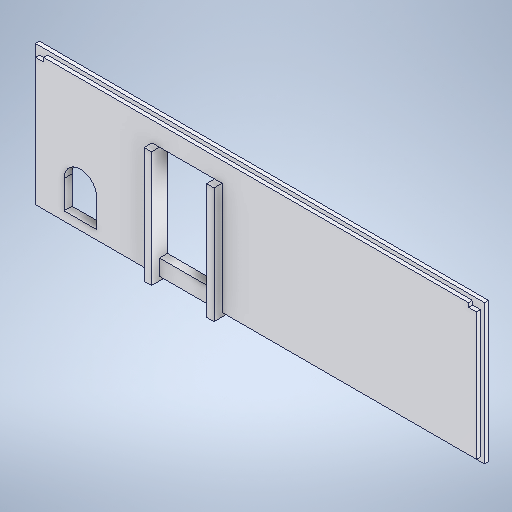
# Autodesk Inventor part: back
Saved by Autodesk Inventor 2025 (Build 290162000, 162)
## iProperties
Created: 2025-05-20
Part Number: back
Material: Generic
Document SubType Name: Modeling
Designer: ethan
Density: 1 g/cm^3
Appearance: PTFE
Author: ethan
Autodesk Inventor part; units mm, degrees
ref_plane "YZ Plane" through (0, 0, 0) normal (1, 0, 0) x (0, 1, 0)
ref_plane "XZ Plane" through (0, 0, 0) normal (0, 1, 0) x (-1, 0, 0)
ref_plane "XY Plane" through (0, 0, 0) normal (0, 0, 1) x (1, 0, 0)
sketch "Sketch1" plane through (0, 0, 0) normal (0, 0, 1) x (1, 0, 0)
  line L0 (0, 0) -> (224.6, 0)
  line L1 (224.6, 0) -> (224.6, 69.85)
  line L2 (224.6, 69.85) -> (0, 69.85)
  line L3 (0, 69.85) -> (0, 0)
  dimension "d0" = 224.6
  dimension "d1" = 69.85
  constraints: 8 end point, 2 parallel, 1 horizontal, 1 perpendicular
  measures "d0" distance of L2.end L1.end
  measures "d1" distance of L1.end L0.end
extrude "Extrusion1" add sketch "Sketch1" along normal blind 2
sketch "Sketch2" plane through (0, 0, 2) normal (0, 0, 1) x (1, 0, 0)
  line L0 (224.6, 0) -> (224.6, 69.85) projected
  line L1 (224.6, 69.85) -> (0, 69.85) projected
  line L2 (0, 69.85) -> (0, 0) projected
  line L3 (0, 0) -> (224.6, 0) projected
  line L4 (2, 67.85) -> (222.6, 67.85)
  line L5 (222.6, 67.85) -> (222.6, 2)
  line L6 (222.6, 2) -> (2, 2)
  line L7 (2, 2) -> (2, 67.85)
  dimension "d4" = 2
  constraints: 8 end point, 3 other
  measures "d4" distance between parallel lines of L1 L4
extrude "Extrusion2" add sketch "Sketch2" along normal blind 2 contours L4 L5 L6 L7
sketch "Sketch3" plane through (0, 0, 4) normal (0, 0, 1) x (1, 0, 0)
  line L0 (2, 2) -> (222.6, 2) construction
  line L1 (222.6, 2) -> (222.6, 67.85) construction
  line L2 (222.6, 67.85) -> (2, 67.85) construction
  line L3 (2, 67.85) -> (2, 2) construction
  line L4 (2, 67.85) -> (6, 67.85)
  line L5 (6, 67.85) -> (6, 65.85)
  line L6 (6, 65.85) -> (2, 65.85)
  line L7 (2, 65.85) -> (2, 67.85)
  line L8 (222.6, 67.85) -> (218.6, 67.85)
  line L9 (218.6, 67.85) -> (218.6, 65.85)
  line L10 (218.6, 65.85) -> (222.6, 65.85)
  line L11 (222.6, 65.85) -> (222.6, 67.85)
  point P0 (0, 0)
  dimension "d7" = 4
  dimension "d8" = 2
  dimension "d9" = 4
  dimension "d10" = 2
  constraints: 16 end point, 4 parallel, 2 horizontal, 2 perpendicular
  measures "d7" distance of L5.end L6.end
  measures "d8" distance of L4.end L5.end
  measures "d9" distance of L10.end L9.end
  measures "d10" distance of L9.end L8.end
extrude "Extrusion3" cut sketch "Sketch3" against normal blind 2
sketch "Sketch4" plane through (0, 0, 4) normal (0, 0, 1) x (1, 0, 0)
  line L0 (6, 67.85) -> (6, 65.85) construction
  line L1 (6, 65.85) -> (2, 65.85) construction
  line L2 (2, 65.85) -> (2, 2) construction
  line L3 (2, 2) -> (222.6, 2) construction
  line L4 (222.6, 2) -> (222.6, 65.85) construction
  line L5 (222.6, 65.85) -> (218.6, 65.85) construction
  line L6 (218.6, 65.85) -> (218.6, 67.85) construction
  line L7 (218.6, 67.85) -> (6, 67.85) construction
  line L8 (2, 2) -> (24.75, 2) construction
  line L9 (24.75, 2) -> (24.75, 13.5) construction
  line L10 (24.75, 13.5) -> (2, 13.5) construction
  line L11 (2, 13.5) -> (2, 2) construction
  line L12 (16.2953, 6.5) -> (32.5453, 6.5)
  line L13 (32.5453, 6.5) -> (32.5453, 20.5)
  line L14 (32.5453, 20.5) -> (16.2953, 20.5)
  line L15 (16.2953, 20.5) -> (16.2953, 6.5)
  line L16 (16.2953, 6.5) -> (32.5453, 20.5) construction
  line L17 (32.5453, 6.5) -> (16.2953, 20.5) construction
  point P0 (0, 0)
  point P1 (24.4203, 13.5)
  dimension "d13" = 22.75
  dimension "d14" = 11.5
  dimension "d15" = 16.25
  dimension "d16" = 14
  constraints: 20 end point, 4 parallel, 2 horizontal, 2 midpoint, 2 perpendicular, 1 point on line
  measures "d13" distance of L10.end L9.end
  measures "d14" distance of L9.end L8.end
  measures "d15" distance of L14.end L13.end
  measures "d16" distance of L13.end L12.end
extrude "Extrusion4" cut sketch "Sketch4" against normal up to surface (4 mm away)
sketch "Sketch5" plane through (0, 0, 4) normal (0, 0, 1) x (1, 0, 0)
  line L0 (32.5453, 20.5) -> (32.5453, 6.5) construction
  line L1 (32.5453, 6.5) -> (16.2953, 6.5) construction
  line L2 (16.2953, 6.5) -> (16.2953, 20.5) construction
  line L3 (16.2953, 20.5) -> (32.5453, 20.5) construction
  line L4 (6, 67.85) -> (6, 65.85) construction
  line L5 (6, 65.85) -> (2, 65.85) construction
  line L6 (2, 65.85) -> (2, 2) construction
  line L7 (2, 2) -> (222.6, 2) construction
  line L8 (222.6, 2) -> (222.6, 65.85) construction
  line L9 (222.6, 65.85) -> (218.6, 65.85) construction
  line L10 (218.6, 65.85) -> (218.6, 67.85) construction
  line L11 (218.6, 67.85) -> (6, 67.85) construction
  line L12 (32.5453, 20.5) -> (77.7953, 20.5) construction
  line L13 (64.0453, 9.925) -> (91.5453, 9.925)
  line L14 (91.5453, 9.925) -> (91.5453, 57.925)
  line L15 (91.5453, 57.925) -> (64.0453, 57.925)
  line L16 (64.0453, 57.925) -> (64.0453, 9.925)
  line L17 (64.0453, 9.925) -> (91.5453, 57.925) construction
  line L18 (91.5453, 9.925) -> (64.0453, 57.925) construction
  line L19 (77.7953, 20.5) -> (77.7953, 33.925) construction
  point P0 (0, 0)
  dimension "d19" = 45.25
  dimension "d20" = 27.5
  dimension "d21" = 48
  constraints: 16 end point, 2 horizontal, 2 midpoint, 2 parallel, 1 perpendicular, 1 vertical
  measures "d19" distance of L0.start L12.end
  measures "d20" distance of L15.end L14.end
  measures "d21" distance of L14.end L13.end
extrude "Extrusion5" cut sketch "Sketch5" against normal up to surface (4 mm away)
sketch "Sketch6" plane through (0, 0, 4) normal (0, 0, 1) x (1, 0, 0)
  line L0 (91.5453, 57.925) -> (91.5453, 9.925) construction
  line L1 (91.5453, 9.925) -> (64.0453, 9.925) construction
  line L2 (64.0453, 9.925) -> (64.0453, 57.925) construction
  line L3 (64.0453, 57.925) -> (91.5453, 57.925) construction
  line L4 (32.5453, 20.5) -> (32.5453, 6.5) construction
  line L5 (32.5453, 6.5) -> (16.2953, 6.5) construction
  line L6 (16.2953, 6.5) -> (16.2953, 20.5) construction
  line L7 (16.2953, 20.5) -> (32.5453, 20.5) construction
  line L8 (6, 67.85) -> (6, 65.85) construction
  line L9 (6, 65.85) -> (2, 65.85) construction
  line L10 (2, 65.85) -> (2, 2) construction
  line L11 (2, 2) -> (222.6, 2) construction
  line L12 (222.6, 2) -> (222.6, 65.85) construction
  line L13 (222.6, 65.85) -> (218.6, 65.85) construction
  line L14 (218.6, 65.85) -> (218.6, 67.85) construction
  line L15 (218.6, 67.85) -> (6, 67.85) construction
  line L16 (0, 0) -> (224.6, 0) construction
  line L17 (64.0453, 0) -> (60.2953, 0) construction
  line L18 (60.2953, 0) -> (60.2953, 57.925) construction
  line L19 (60.2953, 57.925) -> (64.0453, 57.925) construction
  line L20 (64.0453, 57.925) -> (64.0453, 0) construction
  line L21 (91.5453, 57.925) -> (95.2953, 57.925) construction
  line L22 (95.2953, 57.925) -> (95.2953, 0) construction
  line L23 (95.2953, 0) -> (91.5453, 0) construction
  line L24 (91.5453, 0) -> (91.5453, 57.925) construction
  line L25 (60.2953, 57.925) -> (64.0453, 57.925)
  line L26 (64.0453, 57.925) -> (64.0453, 0)
  line L27 (64.0453, 0) -> (60.2953, 0)
  line L28 (60.2953, 0) -> (60.2953, 57.925)
  line L29 (91.5453, 0) -> (95.2953, 0)
  line L30 (95.2953, 0) -> (95.2953, 57.925)
  line L31 (95.2953, 57.925) -> (91.5453, 57.925)
  line L32 (91.5453, 57.925) -> (91.5453, 0)
  line L33 (64.0453, 9.925) -> (64.0453, 57.925) projected
  dimension "d24" = 3.75
  dimension "d25" = 3.75
  constraints: 32 end point, 8 parallel, 4 horizontal, 4 perpendicular, 2 point on line, 1 collinear
  measures "d24" distance of L18.end L19.end
  measures "d25" distance of L22.end L23.end
extrude "Extrusion6" add sketch "Sketch6" along normal blind 4 and the other way blind 2
sketch "Sketch7" plane through (0, 0, 4) normal (0, 0, 1) x (1, 0, 0)
  line L0 (32.5453, 20.5) -> (32.5453, 6.5) construction
  line L1 (32.5453, 6.5) -> (16.2953, 6.5) construction
  line L2 (16.2953, 6.5) -> (16.2953, 20.5) construction
  line L3 (16.2953, 20.5) -> (32.5453, 20.5) construction
  line L4 (91.5453, 57.925) -> (95.2953, 57.925) construction
  line L5 (95.2953, 57.925) -> (95.2953, 2) construction
  line L6 (95.2953, 2) -> (222.6, 2) construction
  line L7 (222.6, 2) -> (222.6, 65.85) construction
  line L8 (222.6, 65.85) -> (218.6, 65.85) construction
  line L9 (218.6, 65.85) -> (218.6, 67.85) construction
  line L10 (218.6, 67.85) -> (6, 67.85) construction
  line L11 (6, 67.85) -> (6, 65.85) construction
  line L12 (6, 65.85) -> (2, 65.85) construction
  line L13 (2, 65.85) -> (2, 2) construction
  line L14 (2, 2) -> (60.2953, 2) construction
  line L15 (60.2953, 2) -> (60.2953, 57.925) construction
  line L16 (60.2953, 57.925) -> (64.0453, 57.925) construction
  line L17 (64.0453, 57.925) -> (91.5453, 57.925) construction
  line L18 (32.5453, 6.5) -> (32.5453, 20.5) projected
  line L19 (32.5453, 20.5) -> (16.2953, 20.5) projected
  arc A0 (32.5453, 20.5) -> (16.2953, 20.5) centre (24.4203, 20.5) ccw
  line L20 (64.0453, 9.925) -> (64.0453, 2) projected
  line L21 (64.0453, 2) -> (91.5453, 2) projected
  line L22 (91.5453, 2) -> (91.5453, 9.925) projected
  line L23 (91.5453, 9.925) -> (64.0453, 9.925) projected
  point P0 (0, 0)
  dimension "d30" = 8.125
  constraints: 2 point on circle, 1 centre point
  measures "d30" radius of A0
extrude "Extrusion7" cut sketch "Sketch7" against normal up to surface (4 mm away) contours L19 A0
body "Solid1"
